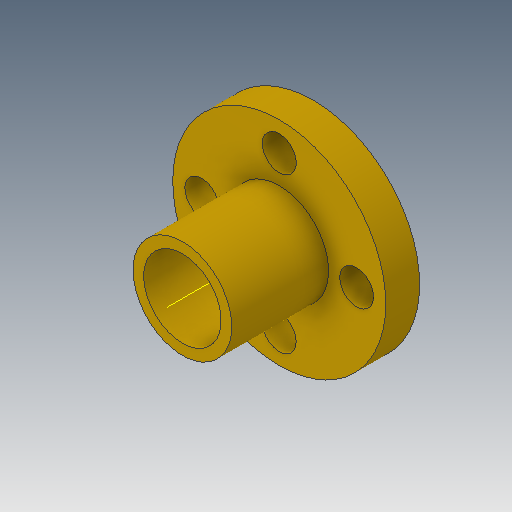
# Autodesk Inventor part: LeadScrewNut
Saved by Autodesk Inventor 2020 (Build 240168000, 168)
## iProperties
Created: 2018-04-20
Part Number: LeadScrewNut
Material: Generic
Document SubType Name: Modeling
Designer: PC  USER
Density: 1 g/cm^3
Appearance: Default
Author: PC  USER
Autodesk Inventor part; units mm, degrees
ref_plane "YZ Plane" through (0, 0, 0) normal (1, 0, 0) x (0, 1, 0)
ref_plane "XZ Plane" through (0, 0, 0) normal (0, 1, 0) x (-1, 0, 0)
ref_plane "XY Plane" through (0, 0, 0) normal (0, 0, 1) x (1, 0, 0)
sketch "Sketch1" plane through (0, 0, 0) normal (1, 0, 0) x (0, 1, 0)
  line L0 (5.1, -7.6) -> (0, -7.6)
  line L1 (0, -7.6) -> (0, 7.6) construction
  line L2 (0, 7.6) -> (5.1, 7.6)
  line L3 (5.1, 7.6) -> (5.1, -7.6)
  line L4 (11, -2.4) -> (5.1, -2.4)
  line L5 (5.1, -2.4) -> (5.1, -5.9)
  line L6 (5.1, -5.9) -> (11, -5.9)
  line L7 (11, -5.9) -> (11, -2.4)
  line L8 (4, 7.6) -> (4, -7.6)
  point P0 (0, 0)
  point P1 (0, 0)
  dimension "d0" = 5.1
  dimension "d1" = 15.2
  dimension "d2" = 3.5
  dimension "d3" = 10
  dimension "d4" = 11
  dimension "d5" = 0
  dimension "d6" = 4
  constraints: 18 end point, 4 parallel, 3 perpendicular, 2 coincident, 2 horizontal, 2 point on line, 1 midpoint
  measures "d0" distance of L1.end L2.end
  measures "d1" distance of L0.end L1.end
  measures "d2" distance of L6.end L4.start
  measures "d3" distance between parallel lines of L4 L2
  measures "d4" distance between parallel lines of L1 L7
  measures "d5" distance between parallel lines of L3 L5
  measures "d6" distance between parallel lines of L1 L8
revolve "Revolution1" add sketch "Sketch1" angle 360 about axis through (0, 0, -7.6) along (0, 0, 1)
sketch "Sketch2" plane through (0, 0, -5.9) normal (0, 0, -1) x (-1, 0, 0)
  circle A0 centre (0, 0) radius 11 projected
  circle A1 centre (0, 0) radius 5.1 projected
  circle A2 centre (0, 8) radius 1.75
  point P0 (0, 0)
  dimension "d8" = 3.5
  dimension "d9" = 8
  constraints: 1 centre point
  measures "d8" diameter of A2
  measures "d9" distance of A2.centre point (0, 0)
extrude "Extrusion1" cut sketch "Sketch2" against normal blind 4 contours A2
pattern_circular "Circular Pattern1" count 4 over 360 about axis through (0, 0, -10) along (0, 0, 1) of "Extrusion1"
body "Solid1"
